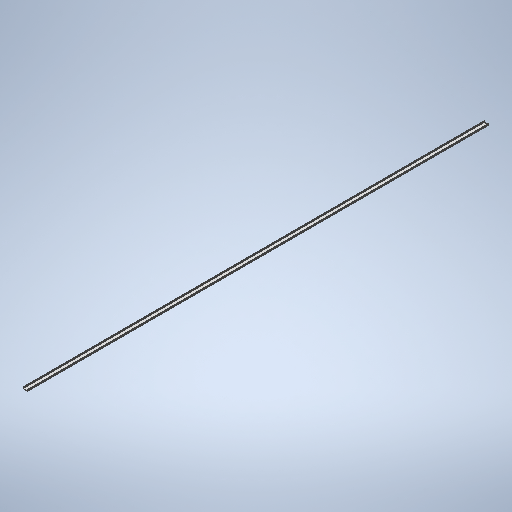
# Autodesk Inventor part: HD - 403 PERFIL ALUMINIO - TRAVESAÑO HORIZONTAL
Saved by Autodesk Inventor 2025 (Build 290162000, 162)
## iProperties
Created: 2026-01-25
Part Number: HD - 403 PERFIL ALUMINIO - TRAVESAÑO HORIZONTAL
Material: Generic
Document SubType Name: Modeling
Designer: Frank
Density: 1 g/cm^3
Appearance: Default
Author: Frank
Autodesk Inventor part; units mm, degrees
ref_plane "YZ Plane" through (0, 0, 0) normal (1, 0, 0) x (0, 1, 0)
ref_plane "XZ Plane" through (0, 0, 0) normal (0, 1, 0) x (-1, 0, 0)
ref_plane "XY Plane" through (0, 0, 0) normal (0, 0, 1) x (1, 0, 0)
sketch "Sketch1" plane through (0, 0, 0) normal (0, 0, 1) x (1, 0, 0)
  line L0 (-2.1658, 15.8) -> (-0.5, 15.8)
  line L1 (0, 15.3) -> (0, 0.5)
  line L2 (-0.5, 0) -> (-25.5, 0)
  line L3 (-3, 2) -> (-25.5, 2)
  line L4 (-25.5, 16.3194) -> (-25.5, -3.3837) construction
  line L5 (-3, 6.6) -> (-5, 6.6)
  line L6 (-5.5, 6.1) -> (-5.5, 5.3)
  line L7 (-5, 4.8) -> (-3, 4.8)
  line L8 (-2.5, 12.0692) -> (-2.5, 7.1)
  line L9 (-2.5, 4.3) -> (-2.5, 2.5)
  line L10 (-3.5088, 13.362) -> (-2.6278, 15.4912)
  line L11 (-3.238, 12.7088) -> (-2.8088, 12.5312)
  arc A0 (-5, 6.6) -> (-5.5, 6.1) centre (-5, 6.1) ccw
  arc A1 (-5.5, 5.3) -> (-5, 4.8) centre (-5, 5.3) ccw
  arc A2 (-2.5, 4.3) -> (-3, 4.8) centre (-3, 4.3) ccw
  arc A3 (-3, 2) -> (-2.5, 2.5) centre (-3, 2.5) ccw
  arc A4 (-0.5, 0) -> (0, 0.5) centre (-0.5, 0.5) ccw
  arc A5 (-3, 6.6) -> (-2.5, 7.1) centre (-3, 7.1) ccw
  arc A6 (-2.5, 12.0692) -> (-2.8088, 12.5312) centre (-3, 12.0692) ccw
  arc A7 (-3.5088, 13.362) -> (-3.238, 12.7088) centre (-3.0468, 13.1708) ccw
  arc A8 (-2.1658, 15.8) -> (-2.6278, 15.4912) centre (-2.1658, 15.3) ccw
  arc A9 (0, 15.3) -> (-0.5, 15.8) centre (-0.5, 15.3) ccw
  line L12 (-48.8342, 15.8) -> (-50.5, 15.8)
  line L13 (-51, 15.3) -> (-51, 0.5)
  line L14 (-50.5, 0) -> (-25.5, 0)
  line L15 (-48, 2) -> (-25.5, 2)
  line L16 (-48, 6.6) -> (-46, 6.6)
  line L17 (-45.5, 6.1) -> (-45.5, 5.3)
  line L18 (-46, 4.8) -> (-48, 4.8)
  line L19 (-48.5, 12.0692) -> (-48.5, 7.1)
  line L20 (-48.5, 4.3) -> (-48.5, 2.5)
  line L21 (-47.4912, 13.362) -> (-48.3722, 15.4912)
  line L22 (-47.762, 12.7088) -> (-48.1912, 12.5312)
  arc A10 (-45.5, 6.1) -> (-46, 6.6) centre (-46, 6.1) ccw
  arc A11 (-46, 4.8) -> (-45.5, 5.3) centre (-46, 5.3) ccw
  arc A12 (-48, 4.8) -> (-48.5, 4.3) centre (-48, 4.3) ccw
  arc A13 (-48.5, 2.5) -> (-48, 2) centre (-48, 2.5) ccw
  arc A14 (-51, 0.5) -> (-50.5, 0) centre (-50.5, 0.5) ccw
  arc A15 (-48.5, 7.1) -> (-48, 6.6) centre (-48, 7.1) ccw
  arc A16 (-48.1912, 12.5312) -> (-48.5, 12.0692) centre (-48, 12.0692) ccw
  arc A17 (-47.762, 12.7088) -> (-47.4912, 13.362) centre (-47.9532, 13.1708) ccw
  arc A18 (-48.3722, 15.4912) -> (-48.8342, 15.8) centre (-48.8342, 15.3) ccw
  arc A19 (-50.5, 15.8) -> (-51, 15.3) centre (-50.5, 15.3) ccw
  point P0 (0, 0)
  point P1 (0, 0)
  point P2 (-5.5, 4.8)
  point P3 (-2.5, 4.8)
  point P4 (-3.7, 12.9)
  point P5 (-2.5, 12.4034)
  point P6 (-51, 0)
  point P7 (-51, 0)
  point P8 (-45.5, 4.8)
  point P9 (-48.5, 4.8)
  point P10 (-47.3, 12.9)
  point P11 (-48.5, 12.4034)
  dimension "d2" = 2
  dimension "d7" = 25.5
  dimension "d10" = 1.8
  dimension "d12" = 15.8
  dimension "d13" = 2.5
  dimension "d14" = 3
  dimension "d15" = 6.3
  dimension "d17" = 1.2
  dimension "d18" = 1.2
  dimension "d19" = 0.5
  constraints: 46 end point, 40 point on circle, 36 symmetric about line, 22 point on line, 20 centre point, 20 tangent, 9 equal radius, 6 perpendicular, 2 coincident, 2 vertical, 1 collinear, 1 horizontal, 1 parallel, 10 other
  measures "d2" distance between parallel lines of L2 L3
  measures "d7" distance between parallel lines of L1 L4
  measures "d10" distance between parallel lines of L5 L7
  measures "d12" distance between parallel lines of L2 L0
  measures "d13" distance between parallel lines of L1 L8
  measures "d14" distance of point (-5.5, 4.8) point (-2.5, 4.8)
  measures "d15" distance from line of L5 point (-3.7, 12.9)
  measures "d17" distance from line of point (-3.7, 12.9) L8
  measures "d18" horizontal distance of point (-2.5, 12.403) point (-3.7, 12.9)
  measures "d19" radius of A0
extrude "Extrusion1" add sketch "Sketch1" against normal blind 5000
body "Solid1"
